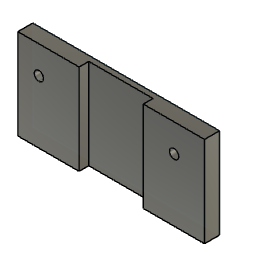
Here3 GPS Link Base Mount (Autodesk Fusion 360 design; units mm, degrees)
Autodesk Fusion 360 part; units mm, degrees
note: some values were not read from the file. Set by a fixed rule: which sketch regions a step uses.
sketch "Sketch1" plane through (0, 0, 0) normal (0, 0, 1) x (1, 0, 0)
  line L0 (0, 0) -> (20.828, 0)
  line L1 (63.5, 0) -> (42.672, 0)
  line L2 (0, 0) -> (0, 5.08)
  line L3 (0, 5.08) -> (20.828, 5.08)
  line L4 (42.672, 5.08) -> (63.5, 5.08)
  line L5 (63.5, 0) -> (63.5, 5.08)
  line L6 (20.828, 0) -> (20.828, 3.2958)
  line L7 (20.828, 3.2958) -> (42.672, 3.2958)
  line L8 (20.828, 5.08) -> (42.672, 5.08)
  line L9 (42.672, 3.2958) -> (42.672, 0)
  constraint coincident L0.start L2.start
  constraint perpendicular L0 L2
  constraint perpendicular L2 L3
  constraint perpendicular L0 L6
  constraint perpendicular L1 L9
extrude "Extrude1" add sketch "Sketch1" along normal blind 26.924
sketch "Sketch2" plane through (0, 5.08, 0) normal (0, 1, 0) x (-1, 0, 0)
  line L0 (0, 0) -> (0, 26.924)
  line L1 (0, 26.924) -> (-63.5, 26.924)
  line L2 (-63.5, 26.924) -> (-63.5, 0)
  circle A0 centre (-7.1438, 17.4625) radius 1.5875
  ellipse E0 centre (-31.75, 10.16) end of major axis (-31.75, 18.415) minor radius 4.445
  line L3 (-27.305, 10.16) -> (-36.195, 10.16)
  spline S0 degree 3 poles (-31.75, 0.1349) (-30.6252, 0.1349) (-29.5498, 0.6153) (-28.7124, 1.3406) (-27.1361, 2.7058) (-26.2, 4.888) (-25.7772, 7.314) (-25.206, 10.5911) (-25.6492, 14.296) (-27.0914, 16.9155) (-27.751, 18.1134) (-28.6277, 19.1179) (-29.7766, 19.7012) (-30.7136, 20.1769) (-31.8485, 20.3138) (-32.8706, 20.0327) (-34.1147, 19.6905) (-35.1265, 18.8268) (-35.8882, 17.7496) (-37.3212, 15.7231) (-38.0067, 12.8125) (-37.9632, 9.9044) (-37.9278, 7.5371) (-37.4042, 5.2029) (-36.3978, 3.385) (-35.7475, 2.2104) (-34.8878, 1.224) (-33.7651, 0.6402) (-33.1503, 0.3205) (-32.4536, 0.1349) (-31.75, 0.1349) knots -3.141593 -3.141593 -3.141593 -3.141593 -2.705208 -2.705208 -2.705208 -1.883824 -1.883824 -1.883824 -0.77427 -0.77427 -0.77427 -0.26685 -0.26685 -0.26685 0.147027 0.147027 0.147027 0.65081 0.65081 0.65081 1.598554 1.598554 1.598554 2.370073 2.370073 2.370073 2.868594 2.868594 2.868594 3.141593 3.141593 3.141593 3.141593
  circle A1 centre (-53.1749, 17.4625) radius 1.5875
  dimension "d20" = 16.51
  dimension "d21" = 8.89
  dimension "d29" = 1.7701
  dimension "d39" = 3.175
  constraint coincident E0 L3.start
  constraint coincident E0 L3.end
  measures "d20" distance of E0
  measures "d39" diameter of A1
extrude "Extrude2" add 1 faces at (56.5573, 2.7919, 0) along direction (0, 0, -1) blind 3.81
sketch "Sketch3" plane through (0, 5.08, 0) normal (0, 1, 0) x (-1, 0, 0)
  line L0 (0, -3.81) -> (0, 26.924)
  line L1 (0, 26.924) -> (-63.5, 26.924)
  line L2 (-63.5, 26.924) -> (-63.5, -3.81)
  line L3 (-63.5, -3.81) -> (0, -3.81)
extrude "Extrude3" cut sketch "Sketch2" against normal blind 7.62 contours A0
sketch "Sketch5" plane through (31.75, 5.08, 11.557) normal (0, 1, 0) x (-1, 0, 0)
  ellipse E0 centre (0, -1.27) end of major axis (0, 6.985) minor radius 4.445
  line L0 (0, -9.525) -> (0, 6.985)
  line L1 (4.445, -1.27) -> (-4.445, -1.27)
  spline S0 degree 3 poles (0, -11.303) (1.1254, -11.303) (2.2015, -10.8229) (3.0394, -10.0983) (4.6119, -8.7385) (5.5474, -6.5684) (5.9741, -4.1542) (6.5537, -0.8752) (6.1164, 2.8385) (4.6769, 5.4685) (4.0195, 6.6695) (3.1454, 7.6778) (1.9981, 8.2674) (1.0631, 8.7479) (-0.0714, 8.8924) (-1.0963, 8.6175) (-2.3365, 8.2847) (-3.3493, 7.433) (-4.1128, 6.3689) (-5.5459, 4.3715) (-6.2416, 1.5015) (-6.2226, -1.3823) (-6.2069, -3.7752) (-5.6923, -6.1456) (-4.685, -7.9935) (-4.0389, -9.1789) (-3.1833, -10.1765) (-2.062, -10.774) (-1.4353, -11.1079) (-0.7215, -11.303) (0, -11.303) knots -3.141593 -3.141593 -3.141593 -3.141593 -2.705795 -2.705795 -2.705795 -1.887989 -1.887989 -1.887989 -0.777204 -0.777204 -0.777204 -0.269962 -0.269962 -0.269962 0.14347 0.14347 0.14347 0.643822 0.643822 0.643822 1.582981 1.582981 1.582981 2.362287 2.362287 2.362287 2.862177 2.862177 2.862177 3.141593 3.141593 3.141593 3.141593
  dimension "d33" = 16.51
  dimension "d34" = 8.89
  dimension "d35" = 1.778
  constraint coincident E0 L0.start
  constraint coincident E0 L0.end
  constraint coincident E0 L1.start
  constraint coincident E0 L1.end
  measures "d33" distance of E0
extrude "Extrude4" add sketch "Sketch5" along normal blind 6.35
extrude "Extrude5" cut sketch "Sketch2" against normal blind 10.16 contours A1
